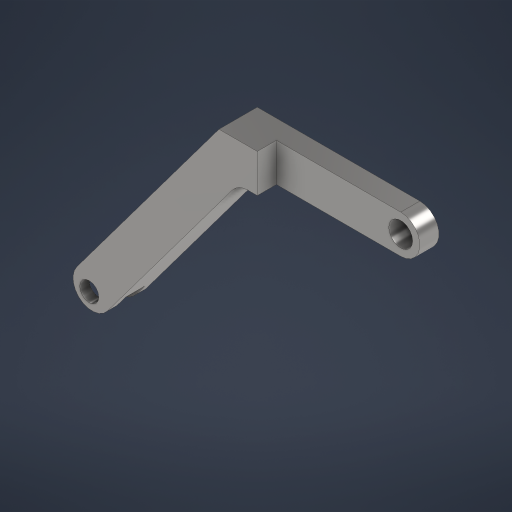
# Autodesk Inventor part: Servo_Strut_v2
Saved by Autodesk Inventor 2023 (Build 270158000, 158)
## iProperties
Created: 2023-02-25
Part Number: Servo_Strut_v2
Material: Steel, Carbon
Document SubType Name: Modeling
Designer: roota
Density: 7.85 g/cm^3
Appearance: Semi-Polished
Mass: 33.4264 g
Surface Area: 27.0753 cm^2
Volume: 4.25814 cm^3
Author: roota
Autodesk Inventor part; units mm, degrees
ref_plane "YZ Plane" through (0, 0, 0) normal (1, 0, 0) x (0, 1, 0)
ref_plane "XZ Plane" through (0, 0, 0) normal (0, 1, 0) x (-1, 0, 0)
ref_plane "XY Plane" through (0, 0, 0) normal (0, 0, 1) x (1, 0, 0)
sketch "Sketch1" plane through (0, 0, 0) normal (0, 0, 1) x (1, 0, 0)
  line L0 (0, 0) -> (-34, 0)
  line L1 (-34, 0) -> (-63.7277, -39.7685)
  line L2 (-63.7277, -39.7685) -> (-70.1353, -34.9787)
  line L3 (-70.1353, -34.9787) -> (-38.008, 8)
  line L4 (-38.008, 8) -> (0, 8)
  line L5 (0, 8) -> (0, 0)
  circle A0 centre (-65.1354, -34.9707) radius 1.5
  circle A1 centre (-4, 4) radius 2.5
  line L6 (0, 4) -> (-36.004, 4) construction
  line L7 (-36.004, 4) -> (-66.9315, -37.3736) construction
  line L8 (0, 0) -> (-63.7277, -39.7685) construction
  dimension "d0" = 8
  dimension "d1" = 3
  dimension "d2" = 5
  dimension "d3" = 4
  dimension "d4" = 3
  dimension "d5" = 72.5
  dimension "d6" = 18
  dimension "d7" = 34
  constraints: 18 end point, 3 perpendicular, 2 centre point, 2 horizontal, 2 midpoint, 2 parallel, 2 point on line, 1 equal length
  measures "d0" distance of L4.end L0.start
  measures "d1" diameter of A0
  measures "d2" diameter of A1
  measures "d3" distance from line of L5 A1.centre
  measures "d4" distance from line of L2 A0.centre
  measures "d5" distance of A1.centre A0.centre
  measures "d6" distance from line of L8 L0.end
  measures "d7" distance of L0.start L0.end
extrude "Extrusion1" add sketch "Sketch1" along normal blind 8
sketch "Sketch2" plane through (-70.1353, -34.9787, 8) normal (-0.8009527, 0.5987276, 0) x (0.5987276, 0.8009527, 0)
  line L0 (0, 8) -> (0, 0) projected
  line L1 (0, 2) -> (7, 2)
  line L2 (7, 2) -> (7, 6)
  line L3 (7, 6) -> (0, 6)
  line L4 (0, 6) -> (0, 2)
  point P0 (70.0082, 8)
  point P1 (0, 6)
  dimension "d10" = 2
  dimension "d11" = 4
  dimension "d13" = 7
  constraints: 8 end point, 2 parallel, 1 horizontal, 1 perpendicular, 1 point on line
  measures "d10" distance from line of L3 L0.start
  measures "d11" distance of L1.end L2.end
  measures "d13" distance of L1.start L1.end
extrude "Extrusion2" cut sketch "Sketch2" against normal blind 8
sketch "Sketch3" plane through (0, 0, 8) normal (0, 0, 1) x (1, 0, 0)
  circle A0 centre (-65.1354, -34.9707) radius 1.5 projected
  circle A1 centre (-65.1354, -34.9707) radius 2
  point P0 (0, 0)
  dimension "d16" = 4
  constraints: 1 centre point, 1 coincident
  measures "d16" diameter of A1
extrude "Extrusion3" cut sketch "Sketch3" against normal up to surface (6 mm away) contours A0 | A1
fillet "Fillet1" radius 4 7 edges at (-70.1353, -34.9787, 7) (-70.1353, -34.9787, 1) (-63.7277, -39.7685, 1) (-63.7277, -39.7685, 7) (0, 8, 4) (0, 0, 4) (-34, 0, 4)
sketch "Sketch4" plane through (0, 0, 8) normal (0, 0, 1) x (1, 0, 0)
  line L0 (0, 0) -> (-30, 0)
  line L1 (-30, 0) -> (-30, 16.3827)
  line L2 (-30, 16.3827) -> (0, 16.3827)
  line L3 (0, 16.3827) -> (0, 0)
  dimension "d20" = 30
  constraints: 8 end point, 2 parallel, 1 coincident, 1 horizontal, 1 perpendicular
  measures "d20" distance of L1.end L2.end
extrude "Extrusion4" cut sketch "Sketch4" against normal blind 4
equation "\"d3\" = 0.5 * d0"
equation "\"d4\" = d1"
body "Solid1"
